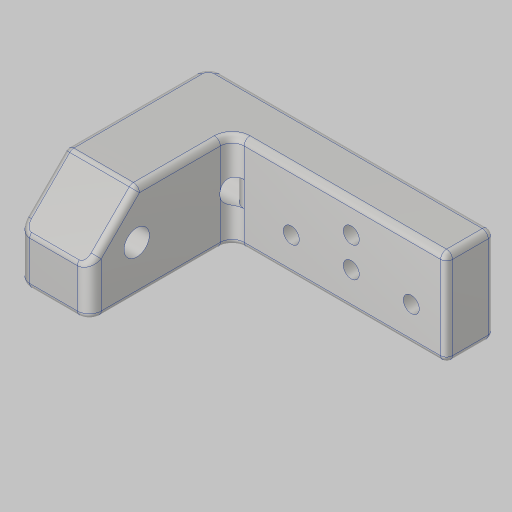
# Autodesk Inventor part: EL2-040
Saved by Autodesk Inventor 2023.5 (Build 275446000, 446)
## iProperties
Created: 2025-02-28
Part Number: EL2-040
Material: Aluminum 6061
Document SubType Name: Modeling
Designer: brand
Density: 2.7 g/cm^3
Appearance: Aluminum - Flat
Author: brand
Autodesk Inventor part; units mm, degrees
ref_plane "YZ Plane" through (0, 0, 0) normal (1, 0, 0) x (0, 1, 0)
ref_plane "XZ Plane" through (0, 0, 0) normal (0, 1, 0) x (-1, 0, 0)
sketch "Sketch1" plane through (0, 0, 0) normal (0, 0, 1) x (1, 0, 0)
  line L0 (-50.8, 15.875) -> (25.4, 15.875)
  line L1 (25.4, 15.875) -> (25.4, -9.525)
  line L2 (25.4, -9.525) -> (-50.8, -9.525)
  line L3 (-50.8, -9.525) -> (-50.8, 15.875)
  point P0 (0, 0)
  point P1 (16, 0)
  point P2 (-16, 0)
  point P3 (0, 8)
  dimension "d0" = 16
  dimension "d1" = 16
  dimension "d4" = 15.875
  dimension "d6" = 76.2
  dimension "d8" = 25.4
  dimension "d44" = 50.8
  dimension "d45" = 9.525
  dimension "d46" = 8
  constraints: 8 end point, 2 horizontal alignment, 2 parallel, 1 horizontal, 1 perpendicular, 1 vertical alignment
  measures "d0" distance of point (0, 0) point (-16, 0)
  measures "d1" distance of point (16, 0) point (0, 0)
  measures "d4" distance from line of L0 point (0, 0)
  measures "d6" distance between parallel lines of L3 L1
  measures "d8" distance of L2.end L0.start
  measures "d44" distance from line of L3 point (0, 8)
  measures "d45" distance from line of L2 point (-16, 0)
  measures "d46" distance of point (0, 0) point (0, 8)
extrude "Extrusion1" add sketch "Sketch1" along normal mid plane 50.8
sketch "Sketch2" plane through (-50.8, -9.525, -25.4) normal (-1, 0, 0) x (0, 0, -1)
  line L0 (-38.1635, -12.7) -> (-12.6365, -12.7) construction
  line L1 (0, -25.4) -> (-50.8, -25.4) construction
  line L2 (0, 0) -> (0, -25.4) construction
  point P0 (-25.4, -9.525)
  point P1 (-25.4, -12.7)
  point P2 (-25.4, -25.4)
  point P3 (0, -12.7)
  dimension "d18" = 25.527
  constraints: 2 end point, 2 midpoint, 1 horizontal, 1 horizontal alignment, 1 vertical alignment, 2 other
  measures "d18" distance of L0.start L0.end
hole "Hole2" at (-50.8, 3.175, -12.7635) at (-50.8, 3.175, 12.7635) direction (1, 0, 0) diameter 6.75 depth 19.05
ref_plane "Work Plane2" through (0, 0, -39.3135) normal (0, 0, -1) x (-1, 0, 0)
ref_plane "Work Plane1" through (0, 0, -95.3135) normal (0, 0, -1) x (-1, 0, 0)
sketch "Sketch3" plane through (-50.8, 15.875, 25.4) normal (0, 1, 0) x (1, 0, 0)
  line L0 (0, 50.8) -> (0, 0) construction
  line L1 (76.2, 0) -> (0, 0) construction
  line L2 (76.2, 50.8) -> (76.2, 0) construction
  line L3 (0, 50.8) -> (76.2, 50.8) construction
  line L4 (76.2, 0) -> (0, 0) construction
  line L5 (9.525, 0) -> (9.525, 50.8) construction
  line L6 (0, 50.8) -> (76.2, 50.8) construction
  line L7 (0, 0) -> (76.2, 0) construction
  line L8 (76.2, 0) -> (19.05, 0)
  line L9 (19.05, 0) -> (19.05, 38.1)
  line L10 (19.05, 38.1) -> (76.2, 38.1)
  line L11 (76.2, 38.1) -> (76.2, 0)
  point P0 (50.8, 25.4)
  dimension "d28" = 9.525
  dimension "d29" = 12.7
  dimension "d30" = 19.05
  constraints: 10 end point, 2 parallel, 2 perpendicular, 2 point on line, 1 horizontal
  measures "d28" distance between parallel lines of L0 L5
  measures "d29" distance between parallel lines of L3 L10
  measures "d30" distance between parallel lines of L0 L9
extrude "Extrusion2" cut sketch "Sketch3" against normal through all
sketch "Sketch4" plane through (-31.75, 15.875, -12.7) normal (0, 0, 1) x (1, 0, 0)
  point P0 (31.75, -15.875)
  point P1 (15.75, -15.875)
  point P2 (31.75, -15.875)
  point P3 (47.75, -15.875)
  point P4 (31.75, -7.875)
hole "Hole3" at (-16, 0, -12.7) at (0, 0, -12.7) at (16, 0, -12.7) at (0, 8, -12.7) direction (0, 0, -1) diameter 4.25 end through all
fillet "Fillet1" radius 3.175 3 edges at (-31.75, 3.175, 25.4) (-50.8, 3.175, 25.4) (-50.8, 3.175, -25.4)
fillet "Fillet3" radius 3.175 3 edges at (-31.75, 11.2122, -12.7) (-31.75, 3.175, -12.7) (-31.75, -4.8622, -12.7)
fillet "Fillet4" radius 1.5875 2 edges at (25.4, 3.175, -12.7) (25.4, 3.175, -25.4)
sketch "Sketch5" plane through (-50.8, -9.525, -22.225) normal (-1, 0, 0) x (0, 0, 1)
  line L0 (0, 0) -> (0, 25.4) construction
  line L1 (44.45, 0) -> (0, 0) construction
  line L2 (44.45, 25.4) -> (44.45, 0) construction
  line L3 (0, 25.4) -> (44.45, 25.4) construction
  circle A0 centre (9.4615, 12.7) radius 3.375 construction
  circle A1 centre (34.9885, 12.7) radius 3.375 construction
  line L4 (47.625, 0) -> (47.625, 25.4) construction
  line L5 (44.45, 0) -> (47.625, 0) construction
  line L6 (47.625, 0) -> (47.625, 25.4) construction
  line L7 (47.625, 25.4) -> (44.45, 25.4) construction
  line L8 (44.45, 25.4) -> (44.45, 0) construction
  line L9 (44.45, 25.4) -> (12.7, 25.4) construction
  line L10 (34.925, 25.4) -> (47.625, 12.7)
  line L11 (47.625, 25.4) -> (47.625, 0) construction
  line L12 (44.45, 25.4) -> (47.625, 25.4) construction
  line L13 (34.925, 25.4) -> (47.625, 25.4)
  line L14 (47.625, 25.4) -> (47.625, 12.7)
  point P0 (22.225, 9.525)
  dimension "d48" = 45
  dimension "d49" = 12.7
  constraints: 6 end point, 1 horizontal, 1 midpoint, 1 perpendicular, 1 point on line
  measures "d48" angle of L10 L3
  measures "d49" distance from line of L4 L10.start
extrude "Extrusion3" cut sketch "Sketch5" against normal through all
fillet "Fillet5" radius 1.5875 27 edges at (-41.275, 15.875, 12.7) (24.935, 15.875, -24.935) (25.4, 15.875, -19.05) (24.935, 15.875, -13.165) (-2.3813, 15.875, -12.7) (-30.8201, 15.875, -11.7701) (-31.75, 15.875, 1.5875) (-49.8701, 15.875, -24.4701) (-50.8, 15.875, -4.7625) (-11.9063, 15.875, -25.4) (-49.8701, -9.525, -24.4701) (-11.9062, -9.525, -25.4) (24.935, -9.525, -24.935) (25.4, -9.525, -19.05) (24.935, -9.525, -13.165) (-2.3813, -9.525, -12.7) (-30.8201, -9.525, -11.7701) (-31.75, -9.525, 6.35) (-32.6799, -9.525, 24.4701) (-41.275, -9.525, 25.4) (-49.8701, -9.525, 24.4701) (-50.8, -9.525, 0) (-49.8701, 4.1049, 24.4701) (-41.275, 3.175, 25.4) (-32.6799, 4.1049, 24.4701) (-31.75, 11.1125, 17.4625) (-50.8, 11.1125, 17.4625)
equation "\"d1\" = d0"
body "Solid1"
